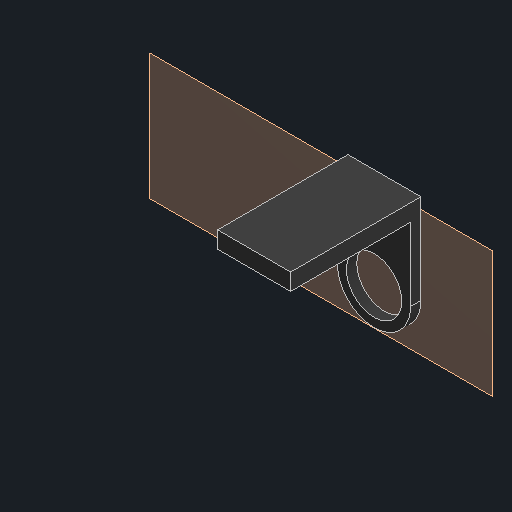
# Autodesk Inventor part: part2
Saved by Autodesk Inventor 2026.1 (Build 301233020, 233B)
## iProperties
Created: 2025-12-10
Part Number: part2
Material: 고무, 검은색
Document SubType Name: Modeling
Designer: jaewook
Density: 0.93 g/cm^3
Appearance: 고무 - 검은색
Author: jaewook
Autodesk Inventor part; units mm, degrees
ref_plane "YZ Plane" through (0, 0, 0) normal (1, 0, 0) x (0, 1, 0)
ref_plane "XZ Plane" through (0, 0, 0) normal (0, 1, 0) x (-1, 0, 0)
ref_plane "XY Plane" through (0, 0, 0) normal (0, 0, 1) x (1, 0, 0)
ref_plane "작업 평면1" through (0, 0, 0) normal (0, 0, 1) x (1, 0, 0)
sketch "스케치1" plane through (0, 0, 0) normal (0, 0, 1) x (1, 0, 0)
  circle A0 centre (28.8901, -8.5) radius 5 projected
  circle A1 centre (28.8901, -8.5) radius 5.3
  circle A2 centre (28.8901, -8.5) radius 7
  line L0 (46.6099, 5.5) -> (-13.1099, 5.5) projected
  line L1 (46.6099, -16.5) -> (46.6099, 5.5) projected
  line L2 (35.8901, -8.5) -> (35.8901, 5.5)
  line L3 (21.8901, -8.5) -> (21.8901, 5.5)
  line L4 (35.8901, 5.5) -> (21.8901, 5.5)
  line L5 (21.8901, 5.5) -> (21.8901, 8.7184)
  line L6 (21.8901, 8.7184) -> (35.8901, 8.7184)
  line L7 (35.8901, 8.7184) -> (35.8901, 5.5)
  line L8 (21.8901, 5.5) -> (35.8901, 5.5)
  point P0 (0, 0)
  point P1 (21.8901, 5.5)
  dimension "d0" = 0.3
  dimension "d1" = 2
  constraints: 14 end point, 3 equal length, 3 perpendicular, 2 centre point, 2 point on circle, 2 point on line, 2 tangent, 1 collinear, 1 horizontal
  measures "d0" radial gap between concentric circles of A0 A1
  measures "d1" radial gap between concentric circles of A0 A2
extrude "돌출1" add sketch "스케치1" along normal blind 2 contours A2 | A2 L3 L0 L2 | L0 L5 L6 L7
sketch "스케치2" plane through (0, 0, 0) normal (0, 0, -1) x (-1, 0, 0)
  line L0 (-21.8901, 8.7184) -> (-21.8901, -8.5) projected
  line L1 (-35.8901, 8.7184) -> (-21.8901, 8.7184) projected
  line L2 (-35.8901, -8.5) -> (-35.8901, 8.7184) projected
  line L3 (13.1099, 5.5) -> (-46.6099, 5.5) projected
  point P0 (0, 0)
  point P1 (-35.8901, 5.5)
  point P2 (-21.8901, 5.5)
extrude "돌출2" add sketch "스케치2" against normal blind 25
